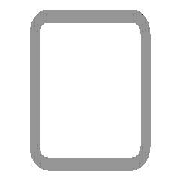
# Autodesk Inventor part: TrägerHöhe1
Saved by Autodesk Inventor 2019.4 (Build 234330000, 330)
## iProperties
IsCustomPart: 1
Created: 2017-10-19
Part Number: TrägerHöhe1
Material: 1.4301
Description: Träger
Document SubType Name: Modeling
Standard: DIN EN 10305-5
Designer: ees GmbH
Standard Revision: 2010-05
Standards Organization: ees
Language: de-DE
Size Designation: 40 x 40 x 1,5  - 2000
Categories: <MemberInstance><Categories><Category DisplayName="Profile" InternalName="089c4875-fa83-4c05-b084-43b9cc11f5ed" Mnemonic="GRDR"><CategoryParameter DisplayName="Masse pro Längeneinheit" InternalName="0bb95a10-148f-4027-a459-38d7b056702a" Mnemonic="shpmass"/><CategoryParameter DisplayName="Querschnittsfläche" InternalName="1ff91680-64b0-4202-b9a3-7fd3f94bba3b" Mnemonic="secarea"/><CategoryParameter DisplayName="Trägheitsradius (x)" InternalName="25778675-03e9-40c1-b6a8-4a9ed693320d" Mnemonic="gyrradx"/><CategoryParameter DisplayName="Torsion-Festigkeitsmodul" InternalName="26c1ec35-5026-4c63-ad0a-751cf684a536" Mnemonic="torrigmod"/><CategoryParameter DisplayName="Abstand zum Schwerpunkt X-X" InternalName="26c9bdb8-9c79-4b4f-a92e-8e197583c9c4" Mnemonic="grcendistX"/><CategoryParameter DisplayName="Alte Varianten-ID" InternalName="340afe4f-75d7-48d3-ab7d-943f3c3da468" Mnemonic="LegacyMemberID"/><CategoryParameter DisplayName="Basislänge" InternalName="42e34263-8f20-4d0e-ad48-bf1385b87c24" Mnemonic="shplen"/><CategoryParameter DisplayName="Trägheitsmoment (y)" InternalName="4b9f58ea-bced-460e-81ea-3d29ca5a49e3" Mnemonic="inermomy"/><CategoryParameter DisplayName="Trägheitsmoment (x)" InternalName="4cd780bc-73d7-43ac-917a-579e5cbd684d" Mnemonic="inermomx"/><CategoryParameter DisplayName="Benutzerdefinierter Basispunkt" InternalName="4f1d1b73-316d-484b-a3df-9cbabb16eb77" Mnemonic="shpBasePoint"/><CategoryParameter DisplayName="Objekthöhe" InternalName="50274e7d-5ac0-4796-92cb-c59e54983c67" Mnemonic="shpheig"/><CategoryParameter DisplayName="Widerstandsmoment (y)" InternalName="59eaa5e9-d227-48dc-b6c1-6920f96e0f95" Mnemonic="secmody"/><CategoryParameter DisplayName="Schnittbezeichnung" InternalName="5a64d034-428d-49c8-ba32-7619764de20f" Mnemonic="shpdes"/><CategoryParameter DisplayName="Widerstandsmoment (x)" InternalName="72cfad18-cf51-4ed4-aaa7-c6b224f8419f" Mnemonic="secmodx"/><CategoryParameter DisplayName="Drehrissmodul" InternalName="7c55a8dc-8844-49f9-a867-cc677b30ec9a" Mnemonic="torsecmod"/><CategoryParameter DisplayName="Objektbreite" InternalName="7c717d54-a18f-4666-b4d4-573cce22c62c" Mnemonic="shpwdth"/><CategoryParameter DisplayName="Zweite Objektdicke" InternalName="9251a8e1-85fd-4e47-af99-afdb762317d9" Mnemonic="shpthick2"/><CategoryParameter DisplayName="GG Erstellt" InternalName="9c666724-f362-4ea7-ac62-f6a007de5c69" Mnemonic="shpFGAuto"/><CategoryParameter DisplayName="Abstand zum Schwerpunkt Y-Y" InternalName="bcc4fb17-7af4-436a-8f8c-d0aa3b0248c5" Mnemonic="grcendistY"/><CategoryParameter DisplayName="Trägheitsradius (y)" InternalName="bfa18ebe-1636-4dbe-8d42-b263e0b73184" Mnemonic="gyrrady"/><CategoryParameter DisplayName="Objektdicke" InternalName="d109cf76-8eb4-42fc-9800-4409734adc67" Mnemonic="shpthick"/><CategoryParameter DisplayName="Koeffizient für Schubverschiebung" InternalName="de4c90c6-aaa8-468f-a335-6737b311b5d3" Mnemonic="shdispc"/><Category DisplayName="Vierkantrohre (quadratisch/rechteckig)" InternalName="afc8e2d8-05d6-4609-8807-f98a9b7d2ed0" Mnemonic="SQRSHP"><CategoryParameter DisplayName="Querschnittsfläche" InternalName="2f7f79dd-983c-4263-802a-5b6a1495fdc5" Mnemonic="secarea"/><CategoryParameter DisplayName="Widerstandsmoment (x)" InternalName="50d965a6-04bf-46b9-8ace-861858d348e6" Mnemonic="secmodx"/><CategoryParameter DisplayName="Widerstandsmoment (y)" InternalName="5106aeac-54a2-4159-a9af-8933dd39dba2" Mnemonic="secmody"/><CategoryParameter DisplayName="Objektdicke" InternalName="52712fc5-f4ee-4eda-b3f2-6fce82c26419" Mnemonic="shpthick"/><CategoryParameter DisplayName="Trägheitsmoment (y)" InternalName="55ec8510-8276-4c45-8f10-594e0fee7eb3" Mnemonic="inermomy"/><CategoryParameter DisplayName="Trägheitsradius (x)" InternalName="56c89926-a299-4389-a862-ac94c9691272" Mnemonic="gyrradx"/><CategoryParameter DisplayName="Radius" InternalName="5d8d062c-e28e-41c1-98da-8e5fee36da1a" Mnemonic="shprad"/><CategoryParameter DisplayName="Trägheitsmoment (x)" InternalName="8c4637b6-6b69-4878-9d5d-26a32185d655" Mnemonic="inermomx"/><CategoryParameter DisplayName="Objektbreite" InternalName="8c8a1782-5e80-4d77-858b-304b1c0ad1fd" Mnemonic="shpwdth"/><CategoryParameter DisplayName="Trägheitsradius (y)" InternalName="fa48a7f5-f030-40f9-a60b-de8a845b7104" Mnemonic="gyrrady"/></Category></Category><Category DisplayName="Datentyp" InternalName="23b78d0f-2648-40c6-8793-ca6db495c9e8" Mnemonic="DATATYPE"><CategoryParameter DisplayName="Anzeigename" InternalName="05415f3d-3907-474b-a020-eb9d644f4cf3" Mnemonic="DISPLAYNAME"/><CategoryParameter DisplayName="Norm" InternalName="0c0a119c-1e12-4c84-803f-101930972f5e" Mnemonic="STANDARD"/><CategoryParameter DisplayName="Beschreibung" InternalName="13903e3d-64b1-4950-80da-f627842ea37f" Mnemonic="DESCRIPTION"/><CategoryParameter DisplayName="Bezeichnung" InternalName="2675968c-4ce5-49e0-a4f5-552d29089031" Mnemonic="DESIGNATION"/><CategoryParameter DisplayName="Standardzeile" InternalName="2af9ec52-faaa-4026-b378-f9fa4afca842" Mnemonic="DEFAULTROW"/><CategoryParameter DisplayName="Ordnername" InternalName="3f06958e-8713-4116-9be7-ed6184ecc97b" Mnemonic="FOLDERNAME"/><CategoryParameter DisplayName="Revisionsanleitung" InternalName="45a75005-10b1-4dfc-8d6d-dfe629f0b93c" Mnemonic="REVISIONGUID"/><CategoryParameter DisplayName="Dateiname" InternalName="8b46a4cc-9585-4fed-90c3-899f57e09a73" Mnemonic="FILENAME"/><CategoryParameter DisplayName="Normungsorganisation" InternalName="8f5914e1-4693-403f-8ab5-d37768198c9d" Mnemonic="STDSORG"/><CategoryParameter DisplayName="Gruppenversion" InternalName="914462f6-6e19-4b14-ba84-155b9680b1d0" Mnemonic="FAMILYREVISION"/><CategoryParameter DisplayName="Normrevision" InternalName="91d5a463-65c2-4fde-b823-3b7fea5e8e17" Mnemonic="STANDARDREVISION"/><CategoryParameter DisplayName="Variantenrevision" InternalName="a65d44b9-392f-4f4f-857b-e4b3d54996fe" Mnemonic="MEMBERREVISION"/><CategoryParameter DisplayName="ClipFormat" InternalName="bc51e27b-3422-4e78-93ef-cec197ddf230" Mnemonic="CLIPFORMAT"/><CategoryParameter DisplayName="Hersteller" InternalName="cd6c7a72-a28a-4e50-99a9-2c7f4e13e5ad" Mnemonic="MANUFACTURER"/><CategoryParameter DisplayName="InternerName" InternalName="cf1d0246-76d9-4b4a-8305-fa0409afb5c1" Mnemonic="INTERNALNAME"/><CategoryParameter DisplayName="IstMetrisch" InternalName="e2385c5b-1ea4-4823-96a8-8de651266ec3" Mnemonic="ISMETRIC"/><Category DisplayName="Bauteil" InternalName="c0e0b642-3bcb-4cc8-9e80-f96d35c4afa4" Mnemonic="PART"><CategoryParameter DisplayName="Bauteilnummer" InternalName="016b6077-bfbe-49bd-92c9-d8d59c39c941" Mnemonic="PARTNUMBER"/><CategoryParameter DisplayName="Bestandsnummer" InternalName="4dba7c1c-e26c-444e-836c-b08b433409a8" Mnemonic="STOCKNUMBER"/><CategoryParameter DisplayName="Materialschlüssel" InternalName="5c9a8adb-dd2b-4535-b97f-0a94a95fe41f" Mnemonic="MATERIALKEY"/><CategoryParameter DisplayName="Material" InternalName="818a152a-d3c3-49ca-80ee-df7d91421b8e" Mnemonic="MATERIAL"/></Category></Category><Category DisplayName="ÄltereVersionenzuweisen" InternalName="cd87c42b-3e48-431e-b5c0-1cbeb14dfe77" Mnemonic="LEGACYMAP"><CategoryParameter DisplayName="Eindeutige DA-Varianten-ID" InternalName="0918ad47-427f-4fed-ae26-24c81c58f590" Mnemonic="DACOOKIE"/><CategoryParameter DisplayName="ID zusammenführen" InternalName="0ee8fb18-e2ed-4f39-96f6-1f4b5f50aa71" Mnemonic="MERGE11"/><CategoryParameter DisplayName="Eindeutige CC-Varianten-ID" InternalName="5193edd4-b2b0-4ab4-9d54-de900eee34e0" Mnemonic="CCCOOKIE"/><CategoryParameter DisplayName="ID aufteilen" InternalName="72b5c83c-be7f-45c4-ae51-9160ea6deb26" Mnemonic="SPLIT"/><CategoryParameter DisplayName="VarianteID" InternalName="8e5e0294-fc51-4c8f-b3d7-003dc5ed94f6" Mnemonic="MEMBERID"/><CategoryParameter DisplayName="Katalogname" InternalName="d99d1e27-aa94-4de2-af4c-c348882a6f4f" Mnemonic="CATALOGNAME"/><CategoryParameter DisplayName="Gruppennummer" InternalName="e705e1f4-09cb-413e-91f9-551b4188271e" Mnemonic="FAMILYNUMBER"/></Category></Categories><FamilyTemplate Id="gp0601"><FamilyTemplateParameters><FamilyTemplateParameter ObjectType="kUserParameterObject" ValueType="xs:double" Id="1" ObjectReferenceKey="G_H"/><FamilyTemplateParameter ObjectType="kUserParameterObject" ValueType="xs:double" Id="2" ObjectReferenceKey="B_L"/><FamilyTemplateParameter ObjectType="kUserParameterObject" ValueType="xs:double" Id="6" ObjectReferenceKey="G_W"/><FamilyTemplateParameter ObjectType="kUserParameterObject" ValueType="xs:double" Id="7" ObjectReferenceKey="G_T"/><FamilyTemplateParameter ObjectType="kUserParameterObject" ValueType="xs:double" Id="8" ObjectReferenceKey="G_IR"/><FamilyTemplateParameter ObjectType="kPropertyObject" ValueType="xs:string" Id="100" ObjectReferenceKey="{32853F0F-3444-11d1-9E93-0060B03C1CA6}" SubObjectId="52"/><FamilyTemplateParameter ObjectType="kPropertyObject" ValueType="xs:string" Id="105" ObjectReferenceKey="{32853F0F-3444-11d1-9E93-0060B03C1CA6}" SubObjectId="5"/><FamilyTemplateParameter ObjectType="kPartComponentDefinitionObject" ValueType="xs:string" Id="110" SubObjectId="Material"/><FamilyTemplateParameter ObjectType="kPropertyObject" ValueType="xs:string" Id="112" ObjectReferenceKey="{32853F0F-3444-11d1-9E93-0060B03C1CA6}" SubObjectId="55"/></FamilyTemplateParameters></FamilyTemplate><CategoryParameterMap><ParamToTemplateMap><ParamToTemplate CategoryParameter="//CategoryParameter[@InternalName='05415f3d-3907-474b-a020-eb9d644f4cf3']" ConstantValue="DIN EN 10305-5 (Geschweißte maßgewalzte Vierkantrohre)"/><ParamToTemplate CategoryParameter="//CategoryParameter[@InternalName='cf1d0246-76d9-4b4a-8305-fa0409afb5c1']" ConstantValue="35e1cc38-09fd-490e-ad4d-98aa2190526a"/><ParamToTemplate CategoryParameter="//CategoryParameter[@InternalName='3f06958e-8713-4116-9be7-ed6184ecc97b']" ConstantValue="DIN EN 10305-5(1)"/><ParamToTemplate CategoryParameter="//CategoryParameter[@InternalName='914462f6-6e19-4b14-ba84-155b9680b1d0']" ConstantValue="10"/><ParamToTemplate CategoryParameter="//CategoryParameter[@InternalName='bc51e27b-3422-4e78-93ef-cec197ddf230']" ConstantValue="CF_INVENTOR.STDPARTS"/><ParamToTemplate CategoryParameter="//CategoryParameter[@InternalName='e2385c5b-1ea4-4823-96a8-8de651266ec3']" ConstantValue="true"/><ParamToTemplate CategoryParameter="//CategoryParameter[@InternalName='13903e3d-64b1-4950-80da-f627842ea37f']" ConstantValue="Präzisionsstahlrohr"/><ParamToTemplate CategoryParameter="//CategoryParameter[@InternalName='8f5914e1-4693-403f-8ab5-d37768198c9d']" ConstantValue="ees"/><ParamToTemplate CategoryParameter="//CategoryParameter[@InternalName='0c0a119c-1e12-4c84-803f-101930972f5e']" ConstantValue="DIN EN 10305-5"/><ParamToTemplate CategoryParameter="//CategoryParameter[@InternalName='cd6c7a72-a28a-4e50-99a9-2c7f4e13e5ad']" TemplateParameter="104"/><ParamToTemplate CategoryParameter="//CategoryParameter[@InternalName='91d5a463-65c2-4fde-b823-3b7fea5e8e17']" ConstantValue="2010-05"/><ParamToTemplate CategoryParameter="//CategoryParameter[@InternalName='45a75005-10b1-4dfc-8d6d-dfe629f0b93c']" ConstantValue="5fbd6c1f-6269-4496-976c-75afc9ff77b2"/><ParamToTemplate CategoryParameter="//CategoryParameter[@InternalName='2af9ec52-faaa-4026-b378-f9fa4afca842']" ConstantValue="1"/><ParamToTemplate CategoryParameter="//CategoryParameter[@InternalName='9c666724-f362-4ea7-ac62-f6a007de5c69']" ConstantValue="1"/><ParamToTemplate CategoryParameter="//CategoryParameter[@InternalName='d99d1e27-aa94-4de2-af4c-c348882a6f4f']" ConstantValue="BSI"/><ParamToTemplate CategoryParameter="//CategoryParameter[@InternalName='e705e1f4-09cb-413e-91f9-551b4188271e']" ConstantValue="158"/><ParamToTemplate CategoryParameter="//CategoryParameter[@InternalName='8b46a4cc-9585-4fed-90c3-899f57e09a73']" ConstantValue="DIN EN 10305-5 - 40 x 40 x 1,5  - 2000"/><ParamToTemplate CategoryParameter="//CategoryParameter[@InternalName='a65d44b9-392f-4f4f-857b-e4b3d54996fe']" ConstantValue="bf1cc477-62ba-45ae-9138-686a849614a8"/><ParamToTemplate CategoryParameter="//CategoryParameter[@InternalName='8c4637b6-6b69-4878-9d5d-26a32185d655']" ConstantValue="5,57"/><ParamToTemplate CategoryParameter="//CategoryParameter[@InternalName='56c89926-a299-4389-a862-ac94c9691272']" ConstantValue="15,5"/><ParamToTemplate CategoryParameter="//CategoryParameter[@InternalName='50d965a6-04bf-46b9-8ace-861858d348e6']" ConstantValue="2,78"/><ParamToTemplate CategoryParameter="//CategoryParameter[@InternalName='2f7f79dd-983c-4263-802a-5b6a1495fdc5']" ConstantValue="2,31"/><ParamToTemplate CategoryParameter="//CategoryParameter[@InternalName='7c55a8dc-8844-49f9-a867-cc677b30ec9a']" ConstantValue="1,81"/><ParamToTemplate CategoryParameter="//CategoryParameter[@InternalName='26c1ec35-5026-4c63-ad0a-751cf684a536']" ConstantValue="4,13"/><ParamToTemplate CategoryParameter="//CategoryParameter[@InternalName='de4c90c6-aaa8-468f-a335-6737b311b5d3']" ConstantValue="2,2807563"/><ParamToTemplate CategoryParameter="//CategoryParameter[@InternalName='5a64d034-428d-49c8-ba32-7619764de20f']" ConstantValue="40 x 40 x 1,5"/><ParamToTemplate CategoryParameter="//CategoryParameter[@InternalName='8e5e0294-fc51-4c8f-b3d7-003dc5ed94f6']" ConstantValue="25"/><ParamToTemplate CategoryParameter="//CategoryParameter[@InternalName='42e34263-8f20-4d0e-ad48-bf1385b87c24']" TemplateParameter="2"/><ParamToTemplate CategoryParameter="//CategoryParameter[@InternalName='2675968c-4ce5-49e0-a4f5-552d29089031']" TemplateParameter="100"/><ParamToTemplate CategoryParameter="//CategoryParameter[@InternalName='50274e7d-5ac0-4796-92cb-c59e54983c67']" TemplateParameter="1"/><ParamToTemplate CategoryParameter="//CategoryParameter[@InternalName='52712fc5-f4ee-4eda-b3f2-6fce82c26419']" TemplateParameter="7"/><ParamToTemplate CategoryParameter="//CategoryParameter[@InternalName='8c8a1782-5e80-4d77-858b-304b1c0ad1fd']" TemplateParameter="6"/><ParamToTemplate CategoryParameter="//CategoryParameter[@InternalName='818a152a-d3c3-49ca-80ee-df7d91421b8e']" TemplateParameter="110"/><ParamToTemplate CategoryParameter="//CategoryParameter[@InternalName='016b6077-bfbe-49bd-92c9-d8d59c39c941']" TemplateParameter="105"/><ParamToTemplate CategoryParameter="//CategoryParameter[@InternalName='4dba7c1c-e26c-444e-836c-b08b433409a8']" TemplateParameter="112"/></ParamToTemplateMap></CategoryParameterMap></MemberInstance>
Stock Number: 2007.003-01.01-101a
Density: 7.9 g/cm^3
Appearance: Halbpoliert(5)
Mass: 1886.44 g
Surface Area: 3193.99 cm^2
Volume: 238.79 cm^3
G_L: 1057,5
Masse: 1.89 kg
Abmessung: =QR <d10> x <d12> - <G_L>
d12: 1,5
d10: 40
Author: ees GmbH
Autodesk Inventor part; units mm, degrees
ref_plane "Startebene" through (0, 0, 0) normal (0, 0, 1) x (1, 0, 0)
ref_plane "Endebene" through (0, 0, 1057.5) normal (0, 0, 1) x (1, 0, 0)
derived "Parameter Skizze.ipt"
sketch "Skizze" plane through (0, 0, 0) normal (0, 0, 1) x (1, 0, 0)
  line L0 (-20, -17.75) -> (-20, 17.75)
  line L1 (-17.75, 20) -> (17.75, 20)
  line L2 (20, 17.75) -> (20, -17.75)
  line L3 (17.75, -20) -> (-17.75, -20)
  arc A0 (-20, -17.75) -> (-17.75, -20) centre (-17.75, -17.75) ccw
  arc A1 (-17.75, 20) -> (-20, 17.75) centre (-17.75, 17.75) ccw
  arc A2 (20, 17.75) -> (17.75, 20) centre (17.75, 17.75) ccw
  arc A3 (17.75, -20) -> (20, -17.75) centre (17.75, -17.75) ccw
  arc A4 (-17.75, 18.5) -> (-18.5, 17.75) centre (-17.75, 17.75) ccw
  line L4 (-17.75, 18.5) -> (17.75, 18.5)
  arc A5 (18.5, 17.75) -> (17.75, 18.5) centre (17.75, 17.75) ccw
  line L5 (18.5, 17.75) -> (18.5, -17.75)
  arc A6 (17.75, -18.5) -> (18.5, -17.75) centre (17.75, -17.75) ccw
  line L6 (17.75, -18.5) -> (-17.75, -18.5)
  arc A7 (-18.5, -17.75) -> (-17.75, -18.5) centre (-17.75, -17.75) ccw
  line L7 (-18.5, -17.75) -> (-18.5, 17.75)
  line L8 (0, 28.6524) -> (0, -28.6524) construction
  line L9 (-28.6524, 0) -> (28.6524, 0) construction
  dimension "d7" = 2.25
  dimension "d10" = 40
  dimension "d11" = 40
  dimension "d12" = 1.5
  dimension "d15" = 20
  dimension "d16" = 20
  constraints: 16 end point, 16 point on circle, 8 centre point, 8 tangent, 4 parallel, 3 equal radius, 2 perpendicular, 7 other
  measures "d7" radius of A0
  measures "d10" distance between parallel lines of L1 L3
  measures "d11" distance between parallel lines of L0 L2
  measures "d12" distance between parallel lines of L2 L5
  measures "d15" distance between parallel lines of L1 L9
  measures "d16" distance between parallel lines of L8 L2
extrude "Körper" add sketch "Skizze" along normal up to surface (1057.5 mm away) from surface at 0
sketch "Sketch3" plane through (0, 0, 0) normal (0, 0, 1) x (1, 0, 0)
  line L0 (0, 0) -> (10, 0)
ref_plane "Work Plane3" through (0, 0, 0) normal (0, -1, 0) x (1, 0, 0)
sketch "Sketch4" plane through (0, 0, 0) normal (0, -1, 0) x (1, 0, 0)
  line L0 (-2, 0) -> (12, 0)
  line L1 (-2, 1057.5) -> (12, 1057.5)
  dimension "d18" = 1057.5
  measures "d18" distance between parallel lines of L0 L1
ref_plane "Arbeitsebene4" through (-17.75, -20, 528.75) normal (0, 0, 1) x (1, 0, 0)
sketch "Skizze9" plane through (17.75, 20, 1057.5) normal (0, 1, 0) x (1, 0, 0)
  line L0 (-31.35, 85.15) -> (-31.35, 124.95)
  line L1 (-31.35, 124.95) -> (-31.35, 434.15) construction
  line L2 (-31.35, 434.15) -> (-31.35, 473.95)
  line L3 (-35.5, 0) -> (0, 0) projected
  line L4 (-37.75, 1057.5) -> (-37.75, 0) projected
  point P0 (-17.75, 1057.5)
  dimension "d77" = 39.8
  dimension "d78" = 85.15
  dimension "d79" = 309.2
  dimension "d80" = 6.4
  constraints: 6 end point, 2 point on line, 1 collinear, 1 vertical
  measures "d77" distance of L0.start L0.end
  measures "d78" distance from line of L0.start L3
  measures "d79" distance of L0.end L1.end
  measures "d80" distance between parallel lines of L0 L4
hole "Bohrung5" [suppressed]
sketch "Skizze10" plane through (-17.75, -20, 0) normal (0, -1, 0) x (1, 0, 0)
  line L0 (37.75, 0) -> (37.75, 1057.5) projected
  line L1 (37.75, 0) -> (37.75, 1057.5) projected
  line L2 (37.75, 0) -> (37.75, 1057.5) projected
  line L3 (37.75, 683) -> (-2.25, 683) construction
  line L4 (35.5, 1057.5) -> (0, 1057.5) projected
  line L5 (-2.25, 0) -> (-2.25, 1057.5) projected
  line L6 (-2.25, 0) -> (-2.25, 1057.5) projected
  point P0 (17.75, 0)
  point P1 (17.75, 683)
  dimension "d91" = 374.5
  constraints: 2 end point, 2 point on line, 1 midpoint, 1 perpendicular
  measures "d91" distance between parallel lines of L3 L4
hole "Bohrung6 Befestigung Seitenhaube" at (0, -20, 683) direction (0, 1, 0) diameter 9 depth 8 tip angle 118 countersink diameter 10 countersink angle 90
pattern_linear "Rechteckige Anordnung1" count 5 spacing 176.875 along (0, 0, 1) of "Bohrung6 Befestigung Seitenhaube" first direction both ways yes
sketch "Skizze11" plane through (-17.75, -20, 0) normal (0, -1, 0) x (1, 0, 0)
  line L0 (35.5, 0) -> (0, 0) projected
  circle A0 centre (17.75, 1036.75) radius 5 projected
  circle A1 centre (17.75, 859.875) radius 5 projected
  circle A2 centre (17.75, 506.125) radius 5 projected
  circle A3 centre (17.75, 329.25) radius 5 projected
  circle A4 centre (17.75, 683) radius 5 projected
  line L1 (35.5, 1057.5) -> (0, 1057.5) projected
  line L2 (0, 0) -> (0, 1057.5) projected
  line L3 (35.5, 0) -> (0, 0) projected
  line L4 (35.5, 0) -> (35.5, 1057.5) projected
  point P0 (17.75, 0)
  point P1 (17.75, 80)
  point P2 (17.75, 228.5)
  point P3 (17.75, 0)
  dimension "d105" = 80
  dimension "d106" = 148.5
  constraints: 2 vertical alignment, 1 midpoint
  measures "d105" distance from line of point (17.75, 80) L0
  measures "d106" distance of point (17.75, 80) point (17.75, 228.5)
hole "Bohrung7 Befestigung Seitenhaube 2" at (0, -20, 80) at (0, -20, 228.5) direction (0, 1, 0) diameter 9 depth 8 tip angle 118 countersink diameter 10 countersink angle 90
sketch "Skizze13" plane through (20, -17.75, 1057.5) normal (1, 0, 0) x (0, 0, -1)
  line L0 (50, 17.75) -> (300, 17.75)
  line L1 (0, 35.5) -> (0, 0) projected
  point P0 (1057.5, 17.75)
  point P1 (0, 17.75)
  dimension "d123" = 50
  dimension "d124" = 250
  constraints: 2 end point, 1 horizontal, 1 horizontal alignment, 1 midpoint
  measures "d123" distance from line of L0.start L1
  measures "d124" distance of L0.start L0.end
hole "Bohrung9 Griff" at (20, 0, 1007.5) at (20, 0, 757.5) direction (-1, 0, 0) diameter 11 depth 8 tip angle 118
sketch "Skizze14" plane through (17.75, 20, 1057.5) normal (0, 1, 0) x (1, 0, 0)
  point P0 (-17.75, 1057.5)
sketch "Skizze15" plane through (-20, 17.75, 0) normal (-1, 0, 0) x (0, 0, 1)
  line L0 (931.5, -7.75) -> (671.5, -7.75)
  line L1 (671.5, -7.75) -> (411.5, -7.75) construction
  line L2 (1057.5, -35.5) -> (1057.5, 0) projected
  line L3 (0, 2.25) -> (1057.5, 2.25) projected
  point P0 (0, -17.75)
  dimension "d132" = 260
  dimension "d133" = 126
  dimension "d141" = 10
  constraints: 4 end point, 1 collinear, 1 horizontal, 1 point on line
  measures "d132" distance of L0.start L0.end
  measures "d133" distance from line of L2 L0.start
  measures "d141" distance between parallel lines of L0 L3
hole "Bohrung10 Leistenbürste" at (-20, 10, 931.5) at (-20, 10, 671.5) at (-20, 10, 411.5) direction (1, 0, 0) diameter 9 depth 8 tip angle 118
sketch "Skizze16" plane through (20, -17.75, 1057.5) normal (1, 0, 0) x (0, 0, -1)
  line L0 (1057.5, 17.75) -> (827.5, 17.75)
  dimension "d142" = 230
  constraints: 2 end point, 1 horizontal
  measures "d142" distance of L0.start L0.end
hole "Bohrung11 Augenschraube" at (20, 0, 230) direction (-1, 0, 0) diameter 11 depth 8 tip angle 118
equation "\"d7\" = rat"
equation "\"d10\" = NMT"
equation "\"d11\" = NMT"
equation "\"d12\" = wst"
equation "\"d15\" = 0.5 * d10"
equation "\"d16\" = 0.5 * d11"
equation "\"d3\" = G_L"
equation "\"G_T\" = 1.5"
equation "\"G_IR\" = 2.25"
equation "\"G_L\" = d18"
equation "\"G_OFFSET_START\" = 0"
equation "\"G_OFFSET_END\" = 0"
equation "\"d14\" = H1"
equation "\"rat\" = 2.25"
equation "\"NMT\" = 40"
equation "\"wst\" = 1.5"
equation "\"H1\" = 1057.5"
body "Solid1"
